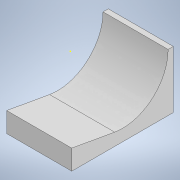
# Autodesk Inventor part: BaseArmHolder
Saved by Autodesk Inventor 2021 (Build 250183000, 183)
## iProperties
Created: 2021-02-21
Part Number: BaseArmHolder
Material: Generic
Document SubType Name: Modeling
Designer: silly
Density: 1 g/cm^3
Appearance: Default
Author: silly
Autodesk Inventor part; units mm, degrees
ref_plane "YZ Plane" through (0, 0, 0) normal (1, 0, 0) x (0, 1, 0)
ref_plane "XZ Plane" through (0, 0, 0) normal (0, 1, 0) x (-1, 0, 0)
ref_plane "XY Plane" through (0, 0, 0) normal (0, 0, 1) x (1, 0, 0)
sketch "Sketch1" plane through (0, 0, 0) normal (1, 0, 0) x (0, 1, 0)
  point P0 (0, 0)
sketch "Sketch2" plane through (0, 0, 0) normal (1, 0, 0) x (0, 1, 0)
  line L0 (-15.1188, 24.4143) -> (6.8812, 24.4143)
  line L1 (6.8812, 24.4143) -> (6.8812, -14.5857)
  line L2 (6.8812, -14.5857) -> (-15.1188, -14.5857)
  line L3 (-15.1188, -14.5857) -> (-15.1188, 24.4143)
  circle A0 centre (6.8812, 4.9143) radius 17.5
  point P0 (0, 0)
  point P1 (6.8812, -12.5857)
  point P2 (6.8812, 22.4143)
  dimension "d0" = 39
  dimension "d1" = 22
  dimension "d2" = 35
  dimension "d5" = 19.5
  dimension "d6" = 19.5
  constraints: 8 end point, 2 parallel, 1 centre point, 1 horizontal, 1 midpoint, 1 perpendicular
  measures "d0" distance between parallel lines of L2 L0
  measures "d1" distance between parallel lines of L3 L1
  measures "d2" diameter of A0
  measures "d5" distance from line of L0 A0.centre
  measures "d6" distance from line of L2 A0.centre
extrude "Extrusion1" add sketch "Sketch2" along normal blind 25 contours L0 L1 A0 L2 L3
sketch "Sketch3" plane through (25, 0, 0) normal (1, 0, 0) x (0, 0, -1)
  arc A0 (-22.4143, 6.8812) -> (12.5857, 6.8812) centre (-4.9143, 6.8812) ccw projected
  line L0 (-4.9143, 6.8812) -> (-7.9532, -10.3529)
  line L1 (-4.9143, 6.8812) -> (12.5857, 6.8812) construction
  line L2 (-7.9532, -10.3529) -> (-24.4143, -7.4504)
  line L3 (-24.4143, 6.8812) -> (-24.4143, -15.1188) projected
  line L4 (-24.4143, -7.4504) -> (-33.9046, 19.8743)
  line L5 (-33.9046, 19.8743) -> (-4.9143, 6.8812)
  point P0 (0, 0)
  dimension "d7" = 100
  constraints: 10 end point, 1 equal length, 1 horizontal, 1 perpendicular, 1 point on circle, 1 point on line
  measures "d7" angle of L0 L1
extrude "Extrusion2" cut sketch "Sketch3" against normal blind 37.625
body "Solid1"
